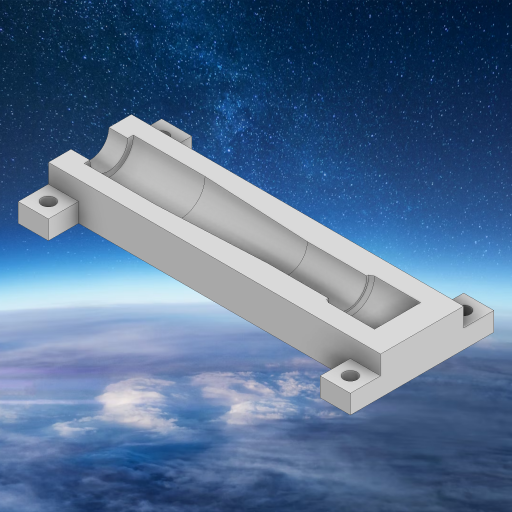
# Autodesk Inventor part: stick_antenna__case_cap
Saved by Autodesk Inventor 2023 (Build 270158000, 158)
## iProperties
Created: 2023-10-30
Part Number: stick_antenna__case_cap
Material: 一般
Document SubType Name: Modeling
Designer: 310611102
Density: 1 g/cm^3
Appearance: 預設
Author: 310611102
Autodesk Inventor part; units mm, degrees
ref_plane "YZ Plane" through (0, 0, 0) normal (1, 0, 0) x (0, 1, 0)
ref_plane "XZ Plane" through (0, 0, 0) normal (0, 1, 0) x (-1, 0, 0)
ref_plane "XY Plane" through (0, 0, 0) normal (0, 0, 1) x (1, 0, 0)
sketch "Sketch1" plane through (0, 0, 0) normal (0, 1, 0) x (-1, 0, 0)
  line L0 (44, 11) -> (-44, 11)
  line L1 (-44, 11) -> (-44, -11)
  line L2 (-44, -11) -> (44, -11)
  line L3 (44, -11) -> (44, 11)
  line L4 (44, 11) -> (-44, -11) construction
  line L5 (-44, 11) -> (44, -11) construction
  line L6 (36, 19) -> (44, 19)
  line L7 (44, 19) -> (44, 11)
  line L8 (44, 11) -> (36, 11)
  line L9 (36, 11) -> (36, 19)
  line L10 (36, 19) -> (44, 11) construction
  line L11 (44, 19) -> (36, 11) construction
  line L12 (36, -19) -> (44, -19)
  line L13 (44, -19) -> (44, -11)
  line L14 (44, -11) -> (36, -11)
  line L15 (36, -11) -> (36, -19)
  line L16 (36, -19) -> (44, -11) construction
  line L17 (44, -19) -> (36, -11) construction
  line L18 (-36, 19) -> (-44, 19)
  line L19 (-44, 19) -> (-44, 11)
  line L20 (-44, 11) -> (-36, 11)
  line L21 (-36, 11) -> (-36, 19)
  line L22 (-36, 19) -> (-44, 11) construction
  line L23 (-44, 19) -> (-36, 11) construction
  line L24 (-36, -19) -> (-44, -19)
  line L25 (-44, -19) -> (-44, -11)
  line L26 (-44, -11) -> (-36, -11)
  line L27 (-36, -11) -> (-36, -19)
  line L28 (-36, -19) -> (-44, -11) construction
  line L29 (-44, -19) -> (-36, -11) construction
  circle A0 centre (40, 15) radius 1.75
  circle A1 centre (40, -15) radius 1.75
  circle A2 centre (-40, 15) radius 1.75
  circle A3 centre (-40, -15) radius 1.75
  point P0 (0, 0)
  dimension "d0" = 22
  dimension "d1" = 88
  dimension "d2" = 8
  dimension "d3" = 8
  dimension "d8" = 3.5
  dimension "d9" = 3.5
  dimension "d10" = 3.5
  dimension "d11" = 3.5
  dimension "d24" = 30
  dimension "d25" = 80
  constraints: 60 end point, 10 midpoint, 10 parallel, 6 equal length, 5 horizontal, 5 perpendicular, 4 centre point, 4 coincident
  measures "d0" distance between parallel lines of L0 L2
  measures "d1" distance of L1.end L2.end
  measures "d2" distance of L6.start L6.end
  measures "d3" distance of L8.end L6.start
  measures "d8" diameter of A0
  measures "d9" diameter of A1
  measures "d10" diameter of A2
  measures "d11" diameter of A3
  measures "d24" distance of point (40, -15) point (40, 15)
  measures "d25" distance of point (-40, 15) point (40, 15)
extrude "Extrusion1" add sketch "Sketch1" along normal blind 10 contours L3 L2 L1 L0
extrude "Extrusion2" add sketch "Sketch1" along normal blind 5 contours L0 L9 L6 L7 | L13 L12 L15 L2 | L0 L19 L18 L21 | L27 L24 L25 L2
sketch "Sketch3" plane through (0, 10, 0) normal (0, 1, 0) x (1, 0, 0)
  line L0 (44, 11) -> (44, 19) projected
  line L1 (-44, -11) -> (44, -11)
  line L2 (44, -11) -> (44, 11)
  line L3 (44, 11) -> (-44, 11)
  line L4 (-44, 11) -> (-44, -11)
  line L5 (-44, -11) -> (44, 11) construction
  line L6 (44, -11) -> (-44, 11) construction
  line L7 (-36, -19) -> (-36, -11) projected
  line L8 (-44, -11) -> (-36, -11) projected
  line L9 (-44, -11) -> (-44, -19) projected
  line L10 (-44, -19) -> (-36, -19) projected
  circle A0 centre (-40, -15) radius 1.75 projected
  line L11 (-36, 11) -> (-44, 11) projected
  line L12 (-36, 11) -> (-36, 19) projected
  line L13 (-36, 19) -> (-44, 19) projected
  line L14 (-44, 19) -> (-44, 11) projected
  circle A1 centre (-40, 15) radius 1.75 projected
  line L15 (36, 19) -> (36, 11) projected
  line L16 (44, 11) -> (36, 11) projected
  line L17 (44, 11) -> (44, 19) projected
  line L18 (44, 19) -> (36, 19) projected
  circle A2 centre (40, 15) radius 1.75 projected
  line L19 (36, -11) -> (44, -11) projected
  line L20 (36, -11) -> (36, -19) projected
  line L21 (36, -19) -> (44, -19) projected
  line L22 (44, -19) -> (44, -11) projected
  circle A3 centre (40, -15) radius 1.75 projected
  point P0 (0, 0)
  constraints: 12 end point, 2 midpoint, 2 parallel, 1 horizontal, 1 perpendicular
sketch "Sketch2" plane through (0, 10, 0) normal (0, 1, 0) x (1, 0, 0)
  line L0 (-98.02, 0) -> (97.5, 0)
  line L1 (-39, 5) -> (-39, 6.5)
  line L2 (-39, 6.5) -> (-20, 6.5)
  line L3 (-20, 6.5) -> (8.5, 5.1)
  line L4 (8.5, 5.1) -> (24.3, 5.1)
  line L5 (24.3, 5.1) -> (24.3, 5.6)
  line L6 (24.3, 5.6) -> (25.3, 6.1)
  line L7 (25.3, 6.1) -> (37.5, 6.1)
  line L8 (37.5, 6.1) -> (37.5, 0)
  line L9 (-38.5, 0) -> (37.5, 0)
  line L10 (-44, 11) -> (-44, -11) projected
  line L11 (-39, 5) -> (-44, 5)
  line L12 (-44, 5) -> (-44, 0)
  point P0 (0, 0)
  dimension "d12" = 13
  dimension "d13" = 12.2
  dimension "d14" = 1
  dimension "d15" = 0.5
  dimension "d16" = 10.2
  dimension "d17" = 76.5
  dimension "d18" = 13.2
  dimension "d19" = 19
  dimension "d20" = 5
  dimension "d21" = 29
  dimension "d23" = 10
  constraints: 24 end point, 4 perpendicular, 4 point on line, 2 parallel, 1 collinear, 1 horizontal, 1 midpoint, 1 vertical
  measures "d12" diameter of L2 L0
  measures "d13" diameter of L7 L0
  measures "d14" distance from line of L6.end L5
  measures "d15" distance of L4.end L5.end
  measures "d16" diameter of L4 L0
  measures "d17" distance between parallel lines of L8 L1
  measures "d18" distance between parallel lines of L8 L5
  measures "d19" distance of L1.end L2.end
  measures "d20" distance between parallel lines of L1 L10
  measures "d21" distance from line of L8 L3.end
  measures "d23" diameter of L11 L0
revolve "Revolution1" cut sketch "Sketch2" angle 360 about axis through (-98.02, 10, 0) along (1, 0, 0)
equation "\"d9\" = d8"
equation "\"d10\" = d8"
equation "\"d11\" = d8"
body "Solid1"
